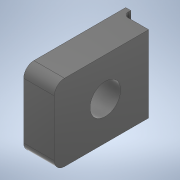
# Autodesk Inventor part: CableHolder
Saved by Autodesk Inventor 2020 (Build 240168000, 168)
## iProperties
Created: 2020-05-24
Part Number: CableHolder
Material: Типовые
Document SubType Name: Modeling
Designer: Михаил
Density: 1 g/cm^3
Appearance: По умолчанию
Author: Михаил
Autodesk Inventor part; units mm, degrees
ref_plane "YZ Plane" through (0, 0, 0) normal (1, 0, 0) x (0, 1, 0)
ref_plane "XZ Plane" through (0, 0, 0) normal (0, 1, 0) x (-1, 0, 0)
ref_plane "XY Plane" through (0, 0, 0) normal (0, 0, 1) x (1, 0, 0)
sketch "Эскиз1" plane through (0, 0, 0) normal (1, 0, 0) x (0, 1, 0)
  line L0 (0, 0) -> (15, 0)
  line L1 (15, 0) -> (15, -20)
  line L2 (15, -20) -> (0, -20)
  line L3 (0, -20) -> (0, 0)
  dimension "d0" = 15
  dimension "d1" = 20
  constraints: 8 end point, 2 parallel, 1 horizontal, 1 perpendicular
  measures "d0" distance of L1.end L2.end
  measures "d1" distance of L0.end L1.end
extrude "Выдавливание1" add sketch "Эскиз1" along normal blind 1
sketch "Эскиз2" plane through (1, 0, 0) normal (1, 0, 0) x (0, 0, -1)
  line L0 (0, 0) -> (20, 0) projected
  line L1 (20, 15) -> (0, 15) projected
  line L2 (0, 0) -> (18.5, 0)
  line L3 (18.5, 0) -> (18.5, 15)
  line L4 (18.5, 15) -> (0, 15)
  line L5 (0, 15) -> (0, 0)
  point P0 (0, 15)
  dimension "d4" = 18.5
  constraints: 8 end point, 2 parallel, 1 horizontal, 1 perpendicular, 1 point on line
  measures "d4" distance of L4.end L3.end
extrude "Выдавливание2" add sketch "Эскиз2" along normal blind 5
sketch "Эскиз3" plane through (0, 0, 0) normal (-1, 0, 0) x (0, 0, 1)
  circle A0 centre (-10, 7.5) radius 3
  line L0 (-20, 0) -> (-20, 15) projected
  line L1 (-20, 15) -> (0, 15) projected
  point P0 (0, 0)
  dimension "d7" = 6
  dimension "d8" = 10
  dimension "d9" = 7.5
  constraints: 1 centre point
  measures "d7" diameter of A0
  measures "d8" distance from line of L0 A0.centre
  measures "d9" distance from line of L1 A0.centre
extrude "Выдавливание3" cut sketch "Эскиз3" against normal blind 10
fillet "Сопряжение1" radius 1 1 edges at (1, 7.5, -18.5)
fillet "Сопряжение2" radius 2 2 edges at (3, 0, 0) (3, 15, 0)
